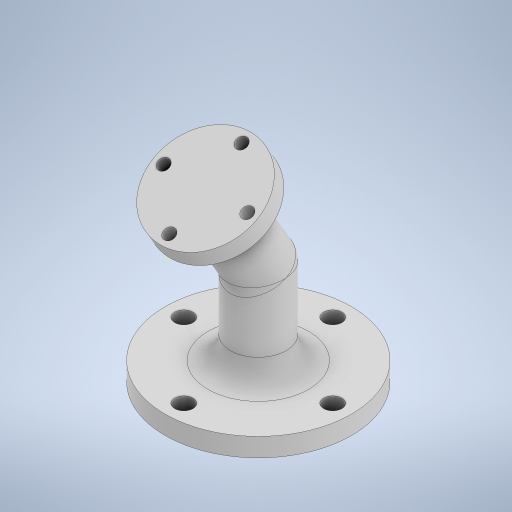
# Autodesk Inventor part: base
Saved by Autodesk Inventor 2023 (Build 270158000, 158)
## iProperties
Created: 2022-11-08
Part Number: base
Material: Genérico
Document SubType Name: Modeling
Designer: Daniel
Density: 1 g/cm^3
Appearance: Valor por defecto
Author: Daniel
Autodesk Inventor part; units mm, degrees
ref_plane "YZ Plane" through (0, 0, 0) normal (1, 0, 0) x (0, 1, 0)
sketch "Boceto1" plane through (0, 0, 0) normal (0, 1, 0) x (-1, 0, 0)
  circle A0 centre (0, 0) radius 25
  dimension "d0" = 50
  constraints: 1 centre point, 1 coincident
  measures "d0" diameter of A0
extrude "Extrusión1" add sketch "Boceto1" along normal blind 5
sketch "Boceto2" plane through (0, 5, 0) normal (0, 1, 0) x (1, 0, 0)
  circle A0 centre (0, 20) radius 2.46
  circle A1 centre (-20, 0) radius 2.46
  circle A2 centre (0, -20) radius 2.46
  circle A3 centre (20, 0) radius 2.46
  point P0 (0, 0)
  dimension "d4" = 4.92
  dimension "d7" = 360
  constraints: 4 centre point, 9 other
  measures "d4" diameter of A0
extrude "Extrusión2" cut sketch "Boceto2" against normal blind 5
sketch "Boceto3" plane through (0, 5, 0) normal (0, 1, 0) x (1, 0, 0)
  circle A0 centre (0, 0) radius 7.5
  dimension "d11" = 15
  constraints: 1 centre point, 1 coincident
  measures "d11" diameter of A0
extrude "Extrusión3" add sketch "Boceto3" along normal blind 25
sketch "Boceto4" plane through (0, 30, 0) normal (0, 1, 0) x (1, 0, 0)
  point P0 (0, 0)
sketch "Boceto5" plane through (0, 30, 0) normal (0, 1, 0) x (1, 0, 0)
  circle A0 centre (0, 0) radius 7.5 projected
  line L0 (0, 0) -> (5.3707, 0)
  line L1 (5.3707, 0) -> (5.3707, 5.235)
  line L2 (5.3707, 5.235) -> (0, 5.235)
  line L3 (0, 5.235) -> (0, 0)
  constraints: 8 end point, 2 parallel, 1 horizontal, 1 perpendicular, 2 other
ref_plane "Plano de trabajo1" through (5.3707, 33.0796, -5.235) normal (0, 0.8619231, 0.507039) x (-1, 0, 0)
sketch "Boceto6" plane through (0, 30, 0) normal (0, 1, 0) x (1, 0, 0)
  circle A0 centre (0, 0) radius 7.5 projected
  line L0 (0, 7.5) -> (-5.4004, 7.5)
  line L1 (-5.4004, 7.5) -> (-5.4004, -0.9159)
  line L2 (-5.4004, -0.9159) -> (0, -0.9159)
  line L3 (0, -0.9159) -> (0, 7.5)
  constraints: 8 end point, 2 parallel, 1 horizontal, 1 perpendicular, 1 vertical alignment, 1 other
ref_plane "Plano de trabajo2" through (0, 30, -7.5) normal (0, 0.8619231, 0.507039) x (-1, 0, 0)
sketch "Boceto7" plane through (0, 30, -7.5) normal (0, 0.8619231, 0.507039) x (-1, 0, 0)
  ellipse E0 centre (0, 6.4644) end of major axis (-7.5, 6.4644) minor radius 6.4644 projected
  line L0 (0, 0) -> (5.4004, 0) projected
  line L1 (0, 7.2538) -> (0, 0) projected
  circle A0 centre (0, 7.5) radius 7.5
  line L2 (0, 0) -> (-6.7565, 0)
  line L3 (0, 0) -> (8.1305, 0)
  point P0 (0, 21.6756)
  point P1 (0, 1.9522)
  dimension "d17" = 15
  constraints: 4 end point, 3 horizontal, 2 vertical alignment, 2 other
extrude "Extrusión5" add sketch "Boceto7" along normal blind 25 contours A0 E0 | A0 E0 picked at (-0.5374, 4.3859) picked at (-0.1044, 14.2669)
delete faces "Suprimir cara1" heal yes whole lump no faces at (-6.1217, 30, -3.9297)
delete faces "Suprimir cara2" heal yes whole lump no faces at (-6.1217, 28.1897, -4.4227)
delete faces "Suprimir cara3" heal yes whole lump no faces at (6.5169, 27.9618, -4.0352)
delete faces "Suprimir cara4" heal yes whole lump no faces at (6.7775, 30, -2.658)
fillet "Empalme2" radius 6 8 edges at (5.3033, 29.4018, -5.3033) (-5.3033, 29.4018, -5.3033) (7.4948, 27.8818, 0.2783) (-7.4948, 27.8818, 0.2783) (-5.4964, 26.568, 5.1029) (-0.5562, 25.9208, 7.4793) (0.5562, 25.9208, 7.4793) (5.4964, 26.568, 5.1029)
fillet "Empalme3" radius 6 1 edges at (-7.5, 5, 0)
sketch "Boceto8" plane through (0, 47.7453, 11.6404) normal (0, 0.8619231, 0.507039) x (1, 0, 0)
  circle A0 centre (0, 0) radius 7.5 projected
  circle A1 centre (0, 0) radius 14
  point P0 (0, -14.1756)
  dimension "d22" = 28
  constraints: 1 centre point, 1 coincident
  measures "d22" diameter of A1
sketch "Boceto9" plane through (0, 47.7453, 11.6404) normal (0, 0.8619231, 0.507039) x (1, 0, 0)
  point P0 (0, -14.1756)
extrude "Extrusión6" add sketch "Boceto8" along normal blind 5 contours A0 | A1
fillet "Empalme4" radius 1 1 edges at (7.5, 47.7453, 11.6404)
sketch "Boceto10" plane through (0, 47.7453, 11.6404) normal (0, -0.8619231, -0.507039) x (1, 0, 0)
  circle A0 centre (0, 0) radius 8.5 projected
  line L0 (8.5, 0) -> (14, 0)
  circle A1 centre (0, 0) radius 14 projected
  circle A2 centre (11.25, 0) radius 1.55
  circle A3 centre (0, 11.25) radius 1.55
  circle A4 centre (-11.25, 0) radius 1.55
  circle A5 centre (0, -11.25) radius 1.55
  point P0 (0, 14.1756)
  dimension "d26" = 3.1
  dimension "d29" = 360
  constraints: 4 centre point, 2 end point, 2 horizontal alignment, 1 horizontal, 1 midpoint, 11 other
  measures "d26" diameter of A2
extrude "Extrusión7" cut sketch "Boceto10" against normal blind 5 contours A2 L0 | L0 A2 | A3 | A4 | A5
